Autodesk Fusion 360 part; units mm, degrees
(part 2 of 3)
extrude "Left inlet bore" cut sketch "Left inlet bore sketch" along normal blind 20.5 bodies 7 in component "06 Gas fitting envelopes TBD"
ref_plane "WorkPlane1" through (0, 0, 3.3) normal (0, 0, 1) x (1, 0, 0) in component "07 Guition 4.3in envelope — depth TBD"
sketch "Guition module envelope sketch" plane through (0, 0, 3.3) normal (0, 0, 1) x (1, 0, 0) in component "07 Guition 4.3in envelope — depth TBD"
  line L0 (-34.705, 10) -> (34.705, 10)
  line L1 (34.705, 10) -> (34.705, 127.01)
  line L2 (34.705, 127.01) -> (-34.705, 127.01)
  line L3 (-34.705, 127.01) -> (-34.705, 10)
  dimension "d549" = 34.705
  dimension "d550" = 10
  dimension "d551" = 69.41
  dimension "d552" = 117.01
  constraint horizontal L0
  constraint vertical L1
  constraint horizontal L2
  constraint vertical L3
  measures "d549" horizontal distance of origin L0.start
  measures "d550" vertical distance of origin L0.start
  measures "d551" horizontal distance of L0.start L0.end
  measures "d552" vertical distance of L0.end L1.end
extrude "Guition module envelope" add sketch "Guition module envelope sketch" along normal blind 13.8 separate body makes body 8 in component "07 Guition 4.3in envelope — depth TBD"
ref_plane "WorkPlane1" through (0, 0, 3.2) normal (0, 0, 1) x (1, 0, 0) in component "08 Active display reference"
sketch "4.3in active screen sketch" plane through (0, 0, 3.2) normal (0, 0, 1) x (1, 0, 0) in component "08 Active display reference"
  line L0 (-28.08, 21.705) -> (28.08, 21.705)
  line L1 (28.08, 21.705) -> (28.08, 115.305)
  line L2 (28.08, 115.305) -> (-28.08, 115.305)
  line L3 (-28.08, 115.305) -> (-28.08, 21.705)
  dimension "d557" = 28.08
  dimension "d558" = 21.705
  dimension "d559" = 56.16
  dimension "d560" = 93.6
  constraint horizontal L0
  constraint vertical L1
  constraint horizontal L2
  constraint vertical L3
  measures "d557" horizontal distance of origin L0.start
  measures "d558" vertical distance of origin L0.start
  measures "d559" horizontal distance of L0.start L0.end
  measures "d560" vertical distance of L0.end L1.end
extrude "4.3in active screen" add sketch "4.3in active screen sketch" along normal blind 0.1 separate body makes body 9 in component "08 Active display reference"
ref_plane "WorkPlane1" through (0, 0, 19) normal (0, 0, 1) x (1, 0, 0) in component "09 Removable electronics carrier"
sketch "Carrier side rail sketch" plane through (0, 0, 19) normal (0, 0, 1) x (1, 0, 0) in component "09 Removable electronics carrier"
  line L0 (-35, 10) -> (-32, 10)
  line L1 (-32, 10) -> (-32, 127)
  line L2 (-32, 127) -> (-35, 127)
  line L3 (-35, 127) -> (-35, 10)
  dimension "d565" = 35
  dimension "d566" = 10
  dimension "d567" = 3
  dimension "d568" = 117
  constraint horizontal L0
  constraint vertical L1
  constraint horizontal L2
  constraint vertical L3
  measures "d565" horizontal distance of origin L0.start
  measures "d566" vertical distance of origin L0.start
  measures "d567" horizontal distance of L0.start L0.end
  measures "d568" vertical distance of L0.end L1.end
extrude "Carrier side rail" add sketch "Carrier side rail sketch" along normal blind 3 separate body makes body 10 in component "09 Removable electronics carrier"
ref_plane "WorkPlane2" through (0, 0, 19) normal (0, 0, 1) x (1, 0, 0) in component "09 Removable electronics carrier"
sketch "Carrier side rail sketch (1)" plane through (0, 0, 19) normal (0, 0, 1) x (1, 0, 0) in component "09 Removable electronics carrier"
  line L0 (32, 10) -> (35, 10)
  line L1 (35, 10) -> (35, 127)
  line L2 (35, 127) -> (32, 127)
  line L3 (32, 127) -> (32, 10)
  dimension "d573" = 32
  dimension "d574" = 10
  dimension "d575" = 3
  dimension "d576" = 117
  constraint horizontal L0
  constraint vertical L1
  constraint horizontal L2
  constraint vertical L3
  measures "d573" horizontal distance of origin L0.start
  measures "d574" vertical distance of origin L0.start
  measures "d575" horizontal distance of L0.start L0.end
  measures "d576" vertical distance of L0.end L1.end
extrude "Carrier side rail (1)" add sketch "Carrier side rail sketch (1)" along normal blind 3 separate body makes body 11 in component "09 Removable electronics carrier"
ref_plane "WorkPlane3" through (0, 0, 19) normal (0, 0, 1) x (1, 0, 0) in component "09 Removable electronics carrier"
sketch "Carrier top crossbar sketch" plane through (0, 0, 19) normal (0, 0, 1) x (1, 0, 0) in component "09 Removable electronics carrier"
  line L0 (-35, 124) -> (35, 124)
  line L1 (35, 124) -> (35, 127)
  line L2 (35, 127) -> (-35, 127)
  line L3 (-35, 127) -> (-35, 124)
  dimension "d581" = 35
  dimension "d582" = 124
  dimension "d583" = 70
  dimension "d584" = 3
  constraint horizontal L0
  constraint vertical L1
  constraint horizontal L2
  constraint vertical L3
  measures "d581" horizontal distance of origin L0.start
  measures "d582" vertical distance of origin L0.start
  measures "d583" horizontal distance of L0.start L0.end
  measures "d584" vertical distance of L0.end L1.end
extrude "Carrier top crossbar" add sketch "Carrier top crossbar sketch" along normal blind 3 bodies 10 11 in component "09 Removable electronics carrier"
ref_plane "WorkPlane4" through (0, 0, 19) normal (0, 0, 1) x (1, 0, 0) in component "09 Removable electronics carrier"
sketch "Carrier middle crossbar sketch" plane through (0, 0, 19) normal (0, 0, 1) x (1, 0, 0) in component "09 Removable electronics carrier"
  line L0 (-35, 87) -> (35, 87)
  line L1 (35, 87) -> (35, 90)
  line L2 (35, 90) -> (-35, 90)
  line L3 (-35, 90) -> (-35, 87)
  dimension "d589" = 35
  dimension "d590" = 87
  dimension "d591" = 70
  dimension "d592" = 3
  constraint horizontal L0
  constraint vertical L1
  constraint horizontal L2
  constraint vertical L3
  measures "d589" horizontal distance of origin L0.start
  measures "d590" vertical distance of origin L0.start
  measures "d591" horizontal distance of L0.start L0.end
  measures "d592" vertical distance of L0.end L1.end
extrude "Carrier middle crossbar" add sketch "Carrier middle crossbar sketch" along normal blind 3 bodies 10 in component "09 Removable electronics carrier"
ref_plane "WorkPlane5" through (0, 0, 19) normal (0, 0, 1) x (1, 0, 0) in component "09 Removable electronics carrier"
sketch "Carrier mounting foot sketch" plane through (0, 0, 19) normal (0, 0, 1) x (1, 0, 0) in component "09 Removable electronics carrier"
  line L0 (-41, 17) -> (-32, 17)
  line L1 (-32, 17) -> (-32, 23)
  line L2 (-32, 23) -> (-41, 23)
  line L3 (-41, 23) -> (-41, 17)
  dimension "d597" = 41
  dimension "d598" = 17
  dimension "d599" = 9
  dimension "d600" = 6
  constraint horizontal L0
  constraint vertical L1
  constraint horizontal L2
  constraint vertical L3
  measures "d597" horizontal distance of origin L0.start
  measures "d598" vertical distance of origin L0.start
  measures "d599" horizontal distance of L0.start L0.end
  measures "d600" vertical distance of L0.end L1.end
extrude "Carrier mounting foot" add sketch "Carrier mounting foot sketch" along normal blind 3 bodies 10 in component "09 Removable electronics carrier"
ref_plane "WorkPlane6" through (0, 0, 18.9) normal (0, 0, 1) x (1, 0, 0) in component "09 Removable electronics carrier"
sketch "Carrier M3 clearance sketch" plane through (0, 0, 18.9) normal (0, 0, 1) x (1, 0, 0) in component "09 Removable electronics carrier"
  circle A0 centre (-38, 20) radius 1.7
  dimension "d605" = 38
  dimension "d606" = 20
  dimension "d607" = 1.7
  measures "d605" horizontal distance of origin A0.centre
  measures "d606" vertical distance of origin A0.centre
  measures "d607" radius of A0
extrude "Carrier M3 clearance" cut sketch "Carrier M3 clearance sketch" along normal blind 3.2 bodies 10 in component "09 Removable electronics carrier"
ref_plane "WorkPlane33" through (0, 0, 3) normal (0, 0, 1) x (1, 0, 0) in component "01 Main housing"
sketch "Carrier support sketch" plane through (0, 0, 3) normal (0, 0, 1) x (1, 0, 0) in component "01 Main housing"
  circle A0 centre (-38, 20) radius 3
  dimension "d612" = 38
  dimension "d613" = 20
  dimension "d614" = 3
  measures "d612" horizontal distance of origin A0.centre
  measures "d613" vertical distance of origin A0.centre
  measures "d614" radius of A0
extrude "Carrier support" add sketch "Carrier support sketch" along normal blind 16 bodies 1 in component "01 Main housing"
ref_plane "WorkPlane34" through (0, 0, 14) normal (0, 0, 1) x (1, 0, 0) in component "01 Main housing"
sketch "Carrier support pilot sketch" plane through (0, 0, 14) normal (0, 0, 1) x (1, 0, 0) in component "01 Main housing"
  circle A0 centre (-38, 20) radius 2.1
  dimension "d619" = 38
  dimension "d620" = 20
  dimension "d621" = 2.1
  measures "d619" horizontal distance of origin A0.centre
  measures "d620" vertical distance of origin A0.centre
  measures "d621" radius of A0
extrude "Carrier support pilot" cut sketch "Carrier support pilot sketch" along normal blind 5.1 bodies 1 in component "01 Main housing"
ref_plane "WorkPlane7" through (0, 0, 19) normal (0, 0, 1) x (1, 0, 0) in component "09 Removable electronics carrier"
sketch "Carrier mounting foot sketch (1)" plane through (0, 0, 19) normal (0, 0, 1) x (1, 0, 0) in component "09 Removable electronics carrier"
  line L0 (-41, 121) -> (-32, 121)
  line L1 (-32, 121) -> (-32, 127)
  line L2 (-32, 127) -> (-41, 127)
  line L3 (-41, 127) -> (-41, 121)
  dimension "d626" = 41
  dimension "d627" = 121
  dimension "d628" = 9
  dimension "d629" = 6
  constraint horizontal L0
  constraint vertical L1
  constraint horizontal L2
  constraint vertical L3
  measures "d626" horizontal distance of origin L0.start
  measures "d627" vertical distance of origin L0.start
  measures "d628" horizontal distance of L0.start L0.end
  measures "d629" vertical distance of L0.end L1.end
extrude "Carrier mounting foot (1)" add sketch "Carrier mounting foot sketch (1)" along normal blind 3 bodies 10 in component "09 Removable electronics carrier"
ref_plane "WorkPlane8" through (0, 0, 18.9) normal (0, 0, 1) x (1, 0, 0) in component "09 Removable electronics carrier"
sketch "Carrier M3 clearance sketch (1)" plane through (0, 0, 18.9) normal (0, 0, 1) x (1, 0, 0) in component "09 Removable electronics carrier"
  circle A0 centre (-38, 124) radius 1.7
  dimension "d634" = 38
  dimension "d635" = 124
  dimension "d636" = 1.7
  measures "d634" horizontal distance of origin A0.centre
  measures "d635" vertical distance of origin A0.centre
  measures "d636" radius of A0
extrude "Carrier M3 clearance (1)" cut sketch "Carrier M3 clearance sketch (1)" along normal blind 3.2 bodies 10 in component "09 Removable electronics carrier"
ref_plane "WorkPlane35" through (0, 0, 3) normal (0, 0, 1) x (1, 0, 0) in component "01 Main housing"
sketch "Carrier support sketch (1)" plane through (0, 0, 3) normal (0, 0, 1) x (1, 0, 0) in component "01 Main housing"
  circle A0 centre (-38, 124) radius 3
  dimension "d641" = 38
  dimension "d642" = 124
  dimension "d643" = 3
  measures "d641" horizontal distance of origin A0.centre
  measures "d642" vertical distance of origin A0.centre
  measures "d643" radius of A0
extrude "Carrier support (1)" add sketch "Carrier support sketch (1)" along normal blind 16 bodies 1 in component "01 Main housing"
ref_plane "WorkPlane36" through (0, 0, 14) normal (0, 0, 1) x (1, 0, 0) in component "01 Main housing"
sketch "Carrier support pilot sketch (1)" plane through (0, 0, 14) normal (0, 0, 1) x (1, 0, 0) in component "01 Main housing"
  circle A0 centre (-38, 124) radius 2.1
  dimension "d648" = 38
  dimension "d649" = 124
  dimension "d650" = 2.1
  measures "d648" horizontal distance of origin A0.centre
  measures "d649" vertical distance of origin A0.centre
  measures "d650" radius of A0
extrude "Carrier support pilot (1)" cut sketch "Carrier support pilot sketch (1)" along normal blind 5.1 bodies 1 in component "01 Main housing"
ref_plane "WorkPlane9" through (0, 0, 19) normal (0, 0, 1) x (1, 0, 0) in component "09 Removable electronics carrier"
sketch "Carrier mounting foot sketch (2)" plane through (0, 0, 19) normal (0, 0, 1) x (1, 0, 0) in component "09 Removable electronics carrier"
  line L0 (32, 17) -> (41, 17)
  line L1 (41, 17) -> (41, 23)
  line L2 (41, 23) -> (32, 23)
  line L3 (32, 23) -> (32, 17)
  dimension "d655" = 32
  dimension "d656" = 17
  dimension "d657" = 9
  dimension "d658" = 6
  constraint horizontal L0
  constraint vertical L1
  constraint horizontal L2
  constraint vertical L3
  measures "d655" horizontal distance of origin L0.start
  measures "d656" vertical distance of origin L0.start
  measures "d657" horizontal distance of L0.start L0.end
  measures "d658" vertical distance of L0.end L1.end
extrude "Carrier mounting foot (2)" add sketch "Carrier mounting foot sketch (2)" along normal blind 3 bodies 10 in component "09 Removable electronics carrier"
ref_plane "WorkPlane10" through (0, 0, 18.9) normal (0, 0, 1) x (1, 0, 0) in component "09 Removable electronics carrier"
sketch "Carrier M3 clearance sketch (2)" plane through (0, 0, 18.9) normal (0, 0, 1) x (1, 0, 0) in component "09 Removable electronics carrier"
  circle A0 centre (38, 20) radius 1.7
  dimension "d663" = 38
  dimension "d664" = 20
  dimension "d665" = 1.7
  measures "d663" horizontal distance of origin A0.centre
  measures "d664" vertical distance of origin A0.centre
  measures "d665" radius of A0
extrude "Carrier M3 clearance (2)" cut sketch "Carrier M3 clearance sketch (2)" along normal blind 3.2 bodies 10 in component "09 Removable electronics carrier"
ref_plane "WorkPlane37" through (0, 0, 3) normal (0, 0, 1) x (1, 0, 0) in component "01 Main housing"
sketch "Carrier support sketch (2)" plane through (0, 0, 3) normal (0, 0, 1) x (1, 0, 0) in component "01 Main housing"
  circle A0 centre (38, 20) radius 3
  dimension "d670" = 38
  dimension "d671" = 20
  dimension "d672" = 3
  measures "d670" horizontal distance of origin A0.centre
  measures "d671" vertical distance of origin A0.centre
  measures "d672" radius of A0
extrude "Carrier support (2)" add sketch "Carrier support sketch (2)" along normal blind 16 bodies 1 in component "01 Main housing"
ref_plane "WorkPlane38" through (0, 0, 14) normal (0, 0, 1) x (1, 0, 0) in component "01 Main housing"
sketch "Carrier support pilot sketch (2)" plane through (0, 0, 14) normal (0, 0, 1) x (1, 0, 0) in component "01 Main housing"
  circle A0 centre (38, 20) radius 2.1
  dimension "d677" = 38
  dimension "d678" = 20
  dimension "d679" = 2.1
  measures "d677" horizontal distance of origin A0.centre
  measures "d678" vertical distance of origin A0.centre
  measures "d679" radius of A0
extrude "Carrier support pilot (2)" cut sketch "Carrier support pilot sketch (2)" along normal blind 5.1 bodies 1 in component "01 Main housing"
ref_plane "WorkPlane11" through (0, 0, 19) normal (0, 0, 1) x (1, 0, 0) in component "09 Removable electronics carrier"
sketch "Carrier mounting foot sketch (3)" plane through (0, 0, 19) normal (0, 0, 1) x (1, 0, 0) in component "09 Removable electronics carrier"
  line L0 (32, 121) -> (41, 121)
  line L1 (41, 121) -> (41, 127)
  line L2 (41, 127) -> (32, 127)
  line L3 (32, 127) -> (32, 121)
  dimension "d684" = 32
  dimension "d685" = 121
  dimension "d686" = 9
  dimension "d687" = 6
  constraint horizontal L0
  constraint vertical L1
  constraint horizontal L2
  constraint vertical L3
  measures "d684" horizontal distance of origin L0.start
  measures "d685" vertical distance of origin L0.start
  measures "d686" horizontal distance of L0.start L0.end
  measures "d687" vertical distance of L0.end L1.end
extrude "Carrier mounting foot (3)" add sketch "Carrier mounting foot sketch (3)" along normal blind 3 bodies 10 in component "09 Removable electronics carrier"
ref_plane "WorkPlane12" through (0, 0, 18.9) normal (0, 0, 1) x (1, 0, 0) in component "09 Removable electronics carrier"
sketch "Carrier M3 clearance sketch (3)" plane through (0, 0, 18.9) normal (0, 0, 1) x (1, 0, 0) in component "09 Removable electronics carrier"
  circle A0 centre (38, 124) radius 1.7
  dimension "d692" = 38
  dimension "d693" = 124
  dimension "d694" = 1.7
  measures "d692" horizontal distance of origin A0.centre
  measures "d693" vertical distance of origin A0.centre
  measures "d694" radius of A0
extrude "Carrier M3 clearance (3)" cut sketch "Carrier M3 clearance sketch (3)" along normal blind 3.2 bodies 10 in component "09 Removable electronics carrier"
ref_plane "WorkPlane39" through (0, 0, 3) normal (0, 0, 1) x (1, 0, 0) in component "01 Main housing"
sketch "Carrier support sketch (3)" plane through (0, 0, 3) normal (0, 0, 1) x (1, 0, 0) in component "01 Main housing"
  circle A0 centre (38, 124) radius 3
  dimension "d699" = 38
  dimension "d700" = 124
  dimension "d701" = 3
  measures "d699" horizontal distance of origin A0.centre
  measures "d700" vertical distance of origin A0.centre
  measures "d701" radius of A0
extrude "Carrier support (3)" add sketch "Carrier support sketch (3)" along normal blind 16 bodies 1 in component "01 Main housing"
ref_plane "WorkPlane40" through (0, 0, 14) normal (0, 0, 1) x (1, 0, 0) in component "01 Main housing"
sketch "Carrier support pilot sketch (3)" plane through (0, 0, 14) normal (0, 0, 1) x (1, 0, 0) in component "01 Main housing"
  circle A0 centre (38, 124) radius 2.1
  dimension "d706" = 38
  dimension "d707" = 124
  dimension "d708" = 2.1
  measures "d706" horizontal distance of origin A0.centre
  measures "d707" vertical distance of origin A0.centre
  measures "d708" radius of A0
extrude "Carrier support pilot (3)" cut sketch "Carrier support pilot sketch (3)" along normal blind 5.1 bodies 1 in component "01 Main housing"
ref_plane "WorkPlane1" through (0, 0, 23) normal (0, 0, 1) x (1, 0, 0) in component "10 Future PCB and component envelope TBD"
sketch "Sketch1 (2)" plane through (0, 0, 23) normal (0, 0, 1) x (1, 0, 0) in component "10 Future PCB and component envelope TBD"
  line L0 (-32, 14) -> (32, 14)
  line L1 (32, 14) -> (32, 122)
  line L2 (32, 122) -> (-32, 122)
  line L3 (-32, 122) -> (-32, 14)
  dimension "d713" = 32
  dimension "d714" = 14
  dimension "d715" = 64
  dimension "d716" = 108
  constraint horizontal L0
  constraint vertical L1
  constraint horizontal L2
  constraint vertical L3
  measures "d713" horizontal distance of origin L0.start
  measures "d714" vertical distance of origin L0.start
  measures "d715" horizontal distance of L0.start L0.end
  measures "d716" vertical distance of L0.end L1.end
extrude "Future PCB envelope — not routed KiCad board" add sketch "Sketch1 (2)" along normal blind 1.6 separate body makes body 12 in component "10 Future PCB and component envelope TBD"
ref_plane "WorkPlane2" through (0, 0, 18.5) normal (0, 0, 1) x (1, 0, 0) in component "10 Future PCB and component envelope TBD"
sketch "Lower PCB component allowance sketch" plane through (0, 0, 18.5) normal (0, 0, 1) x (1, 0, 0) in component "10 Future PCB and component envelope TBD"
  line L0 (-27, 18) -> (27, 18)
  line L1 (27, 18) -> (27, 84)
  line L2 (27, 84) -> (-27, 84)
  line L3 (-27, 84) -> (-27, 18)
  dimension "d721" = 27
  dimension "d722" = 18
  dimension "d723" = 54
  dimension "d724" = 66
  constraint horizontal L0
  constraint vertical L1
  constraint horizontal L2
  constraint vertical L3
  measures "d721" horizontal distance of origin L0.start
  measures "d722" vertical distance of origin L0.start
  measures "d723" horizontal distance of L0.start L0.end
  measures "d724" vertical distance of L0.end L1.end
extrude "Lower PCB component allowance" add sketch "Lower PCB component allowance sketch" along normal blind 4.5 separate body makes body 13 in component "10 Future PCB and component envelope TBD"
ref_plane "WorkPlane3" through (0, 0, 18.5) normal (0, 0, 1) x (1, 0, 0) in component "10 Future PCB and component envelope TBD"
sketch "Upper PCB component allowance sketch" plane through (0, 0, 18.5) normal (0, 0, 1) x (1, 0, 0) in component "10 Future PCB and component envelope TBD"
  line L0 (-27, 93) -> (27, 93)
  line L1 (27, 93) -> (27, 121)
  line L2 (27, 121) -> (-27, 121)
  line L3 (-27, 121) -> (-27, 93)
  dimension "d729" = 27
  dimension "d730" = 93
  dimension "d731" = 54
  dimension "d732" = 28
  constraint horizontal L0
  constraint vertical L1
  constraint horizontal L2
  constraint vertical L3
  measures "d729" horizontal distance of origin L0.start
  measures "d730" vertical distance of origin L0.start
  measures "d731" horizontal distance of L0.start L0.end
  measures "d732" vertical distance of L0.end L1.end
extrude "Upper PCB component allowance" add sketch "Upper PCB component allowance sketch" along normal blind 4.5 separate body makes body 14 in component "10 Future PCB and component envelope TBD"
ref_plane "WorkPlane1" through (0, 0, 27) normal (0, 0, 1) x (1, 0, 0) in component "11 Protected FMA holder envelope TBD"
sketch "FMA holder envelope TBD sketch" plane through (0, 0, 27) normal (0, 0, 1) x (1, 0, 0) in component "11 Protected FMA holder envelope TBD"
  line L0 (-22, 12) -> (22, 12)
  line L1 (22, 12) -> (22, 88)
  line L2 (22, 88) -> (-22, 88)
  line L3 (-22, 88) -> (-22, 12)
  dimension "d737" = 22
  dimension "d738" = 12
  dimension "d739" = 44
  dimension "d740" = 76
  constraint horizontal L0
  constraint vertical L1
  constraint horizontal L2
  constraint vertical L3
  measures "d737" horizontal distance of origin L0.start
  measures "d738" vertical distance of origin L0.start
  measures "d739" horizontal distance of L0.start L0.end
  measures "d740" vertical distance of L0.end L1.end
extrude "FMA holder envelope TBD" add sketch "FMA holder envelope TBD sketch" along normal blind 28 separate body makes body 15 in component "11 Protected FMA holder envelope TBD"
ref_plane "WorkPlane2" through (0, 0, 29) normal (0, 0, 1) x (1, 0, 0) in component "11 Protected FMA holder envelope TBD"
sketch "Two-cell cavity envelope sketch" plane through (0, 0, 29) normal (0, 0, 1) x (1, 0, 0) in component "11 Protected FMA holder envelope TBD"
  line L0 (-20, 16) -> (20, 16)
  line L1 (20, 16) -> (20, 84)
  line L2 (20, 84) -> (-20, 84)
  line L3 (-20, 84) -> (-20, 16)
  dimension "d745" = 20
  dimension "d746" = 16
  dimension "d747" = 40
  dimension "d748" = 68
  constraint horizontal L0
  constraint vertical L1
  constraint horizontal L2
  constraint vertical L3
  measures "d745" horizontal distance of origin L0.start
  measures "d746" vertical distance of origin L0.start
  measures "d747" horizontal distance of L0.start L0.end
  measures "d748" vertical distance of L0.end L1.end
extrude "Two-cell cavity envelope" cut sketch "Two-cell cavity envelope sketch" along normal blind 27 bodies 15 in component "11 Protected FMA holder envelope TBD"
ref_plane "WorkPlane1" through (0, 17, 0) normal (0, 1, 0) x (0, 0, 1) in component "12 Two 18650 cell envelopes"
sketch "18650 envelope" plane through (0, 17, 0) normal (0, 1, 0) x (1, 0, 0) in component "12 Two 18650 cell envelopes"
  circle A0 centre (-10, -39) radius 9.3
  dimension "d753" = 10
  dimension "d754" = 39
  dimension "d755" = 9.3
  measures "d753" horizontal distance of origin A0.centre
  measures "d754" vertical distance of origin A0.centre
  measures "d755" radius of A0
extrude "18650 cell envelope" add sketch "18650 envelope" along normal blind 65.5 separate body makes body 16 in component "12 Two 18650 cell envelopes"
ref_plane "WorkPlane2" through (0, 17, 0) normal (0, 1, 0) x (0, 0, 1) in component "12 Two 18650 cell envelopes"
sketch "18650 envelope (1)" plane through (0, 17, 0) normal (0, 1, 0) x (1, 0, 0) in component "12 Two 18650 cell envelopes"
  circle A0 centre (10, -39) radius 9.3
  dimension "d760" = 10
  dimension "d761" = 39
  dimension "d762" = 9.3
  measures "d760" horizontal distance of origin A0.centre
  measures "d761" vertical distance of origin A0.centre
  measures "d762" radius of A0
extrude "18650 cell envelope (1)" add sketch "18650 envelope (1)" along normal blind 65.5 separate body makes body 17 in component "12 Two 18650 cell envelopes"
ref_plane "WorkPlane1" through (0, 0, 38) normal (0, 0, 1) x (1, 0, 0) in component "13 Battery plug and cable clearance TBD"
sketch "RCY BEC disconnect clearance sketch" plane through (0, 0, 38) normal (0, 0, 1) x (1, 0, 0) in component "13 Battery plug and cable clearance TBD"
  line L0 (23, 18) -> (33, 18)
  line L1 (33, 18) -> (33, 40)
  line L2 (33, 40) -> (23, 40)
  line L3 (23, 40) -> (23, 18)
  dimension "d767" = 23
  dimension "d768" = 18
  dimension "d769" = 10
  dimension "d770" = 22
  constraint horizontal L0
  constraint vertical L1
  constraint horizontal L2
  constraint vertical L3
  measures "d767" horizontal distance of origin L0.start
  measures "d768" vertical distance of origin L0.start
  measures "d769" horizontal distance of L0.start L0.end
  measures "d770" vertical distance of L0.end L1.end
extrude "RCY BEC disconnect clearance" add sketch "RCY BEC disconnect clearance sketch" along normal blind 14 separate body makes body 18 in component "13 Battery plug and cable clearance TBD"
ref_plane "WorkPlane1" through (44.5, 0, 0) normal (1, 0, 0) x (0, 1, 0) in component "14 Supported USB-C mounting insert TBD"
sketch "Replaceable USB insert sketch" plane through (44.5, 0, 0) normal (1, 0, 0) x (0, 0, -1) in component "14 Supported USB-C mounting insert TBD"
  line L0 (-41.75, 58.25) -> (-26.25, 58.25)
  line L1 (-26.25, 58.25) -> (-26.25, 77.75)
  line L2 (-26.25, 77.75) -> (-41.75, 77.75)
  line L3 (-41.75, 77.75) -> (-41.75, 58.25)
  dimension "d775" = 41.75
  dimension "d776" = 58.25
  dimension "d777" = 15.5
  dimension "d778" = 19.5
  constraint horizontal L0
  constraint vertical L1
  constraint horizontal L2
  constraint vertical L3
  measures "d775" horizontal distance of origin L0.start
  measures "d776" vertical distance of origin L0.start
  measures "d777" horizontal distance of L0.start L0.end
  measures "d778" vertical distance of L0.end L1.end
extrude "Replaceable USB insert" add sketch "Replaceable USB insert sketch" along normal blind 3 separate body makes body 19 in component "14 Supported USB-C mounting insert TBD"
ref_plane "WorkPlane2" through (42.5, 0, 0) normal (1, 0, 0) x (0, 1, 0) in component "14 Supported USB-C mounting insert TBD"
sketch "USB interior backing flange sketch" plane through (42.5, 0, 0) normal (1, 0, 0) x (0, 0, -1) in component "14 Supported USB-C mounting insert TBD"
  line L0 (-44, 56) -> (-24, 56)
  line L1 (-24, 56) -> (-24, 80)
  line L2 (-24, 80) -> (-44, 80)
  line L3 (-44, 80) -> (-44, 56)
  dimension "d783" = 44
  dimension "d784" = 56
  dimension "d785" = 20
  dimension "d786" = 24
  constraint horizontal L0
  constraint vertical L1
  constraint horizontal L2
  constraint vertical L3
  measures "d783" horizontal distance of origin L0.start
  measures "d784" vertical distance of origin L0.start
  measures "d785" horizontal distance of L0.start L0.end
  measures "d786" vertical distance of L0.end L1.end
extrude "USB interior backing flange" add sketch "USB interior backing flange sketch" along normal blind 2 separate body makes body 20 in component "14 Supported USB-C mounting insert TBD"
ref_plane "WorkPlane3" through (42.4, 0, 0) normal (1, 0, 0) x (0, 1, 0) in component "14 Supported USB-C mounting insert TBD"
sketch "Sketch3 (2)" plane through (42.4, 0, 0) normal (1, 0, 0) x (0, 0, -1) in component "14 Supported USB-C mounting insert TBD"
  line L0 (-35.93, 63.18) -> (-32.07, 63.18)
  line L1 (-32.07, 63.18) -> (-32.07, 72.82)
  line L2 (-32.07, 72.82) -> (-35.93, 72.82)
  line L3 (-35.93, 72.82) -> (-35.93, 63.18)
  dimension "d791" = 35.93
  dimension "d792" = 63.18
  dimension "d793" = 3.86
  dimension "d794" = 9.64
  constraint horizontal L0
  constraint vertical L1
  constraint horizontal L2
  constraint vertical L3
  measures "d791" horizontal distance of origin L0.start
  measures "d792" vertical distance of origin L0.start
  measures "d793" horizontal distance of L0.start L0.end
  measures "d794" vertical distance of L0.end L1.end
extrude "USB aperture envelope — GCT step profile TBD" cut sketch "Sketch3 (2)" along normal blind 5.2 bodies 19 in component "14 Supported USB-C mounting insert TBD"
ref_plane "WorkPlane4" through (42.4, 0, 0) normal (1, 0, 0) x (0, 1, 0) in component "14 Supported USB-C mounting insert TBD"
sketch "USB backing aperture sketch" plane through (42.4, 0, 0) normal (1, 0, 0) x (0, 0, -1) in component "14 Supported USB-C mounting insert TBD"
  line L0 (-35.93, 63.18) -> (-32.07, 63.18)
  line L1 (-32.07, 63.18) -> (-32.07, 72.82)
  line L2 (-32.07, 72.82) -> (-35.93, 72.82)
  line L3 (-35.93, 72.82) -> (-35.93, 63.18)
  dimension "d799" = 35.93
  dimension "d800" = 63.18
  dimension "d801" = 3.86
  dimension "d802" = 9.64
  constraint horizontal L0
  constraint vertical L1
  constraint horizontal L2
  constraint vertical L3
  measures "d799" horizontal distance of origin L0.start
  measures "d800" vertical distance of origin L0.start
  measures "d801" horizontal distance of L0.start L0.end
  measures "d802" vertical distance of L0.end L1.end
extrude "USB backing aperture" cut sketch "USB backing aperture sketch" along normal blind 2.2 bodies 20 in component "14 Supported USB-C mounting insert TBD"
ref_plane "WorkPlane1" through (0, 0, 33.7) normal (0, 0, 1) x (1, 0, 0) in component "15 USB daughterboard envelope 0.60mm"
sketch "Sketch1 (3)" plane through (0, 0, 33.7) normal (0, 0, 1) x (1, 0, 0) in component "15 USB daughterboard envelope 0.60mm"
  line L0 (29, 60) -> (41, 60)
  line L1 (41, 60) -> (41, 76)
  line L2 (41, 76) -> (29, 76)
  line L3 (29, 76) -> (29, 60)
  dimension "d807" = 29
  dimension "d808" = 60
  dimension "d809" = 12
  dimension "d810" = 16
  constraint horizontal L0
  constraint vertical L1
  constraint horizontal L2
  constraint vertical L3
  measures "d807" horizontal distance of origin L0.start
  measures "d808" vertical distance of origin L0.start
  measures "d809" horizontal distance of L0.start L0.end
  measures "d810" vertical distance of L0.end L1.end
extrude "USB daughterboard — layout TBD" add sketch "Sketch1 (3)" along normal blind 0.6 separate body makes body 21 in component "15 USB daughterboard envelope 0.60mm"
ref_plane "WorkPlane2" through (0, 0, 32.5) normal (0, 0, 1) x (1, 0, 0) in component "15 USB daughterboard envelope 0.60mm"
sketch "GCT connector envelope TBD sketch" plane through (0, 0, 32.5) normal (0, 0, 1) x (1, 0, 0) in component "15 USB daughterboard envelope 0.60mm"
  line L0 (34, 63.5) -> (47.5, 63.5)
  line L1 (47.5, 63.5) -> (47.5, 72.5)
  line L2 (47.5, 72.5) -> (34, 72.5)
  line L3 (34, 72.5) -> (34, 63.5)
  dimension "d815" = 34
  dimension "d816" = 63.5
  dimension "d817" = 13.5
  dimension "d818" = 9
  constraint horizontal L0
  constraint vertical L1
  constraint horizontal L2
  constraint vertical L3
  measures "d815" horizontal distance of origin L0.start
  measures "d816" vertical distance of origin L0.start
  measures "d817" horizontal distance of L0.start L0.end
  measures "d818" vertical distance of L0.end L1.end
extrude "GCT connector envelope TBD" add sketch "GCT connector envelope TBD sketch" along normal blind 3 separate body makes body 22 in component "15 USB daughterboard envelope 0.60mm"
ref_plane "WorkPlane5" through (0, 0, 31.7) normal (0, 0, 1) x (1, 0, 0) in component "14 Supported USB-C mounting insert TBD"
sketch "USB board support ledge sketch" plane through (0, 0, 31.7) normal (0, 0, 1) x (1, 0, 0) in component "14 Supported USB-C mounting insert TBD"
  line L0 (29, 60) -> (42.5, 60)
  line L1 (42.5, 60) -> (42.5, 62)
  line L2 (42.5, 62) -> (29, 62)
  line L3 (29, 62) -> (29, 60)
  dimension "d823" = 29
  dimension "d824" = 60
  dimension "d825" = 13.5
  dimension "d826" = 2
  constraint horizontal L0
  constraint vertical L1
  constraint horizontal L2
  constraint vertical L3
  measures "d823" horizontal distance of origin L0.start
  measures "d824" vertical distance of origin L0.start
  measures "d825" horizontal distance of L0.start L0.end
  measures "d826" vertical distance of L0.end L1.end
extrude "USB board support ledge" add sketch "USB board support ledge sketch" along normal blind 2 separate body makes body 23 in component "14 Supported USB-C mounting insert TBD"
ref_plane "WorkPlane6" through (0, 0, 31.7) normal (0, 0, 1) x (1, 0, 0) in component "14 Supported USB-C mounting insert TBD"
sketch "USB board support ledge sketch (1)" plane through (0, 0, 31.7) normal (0, 0, 1) x (1, 0, 0) in component "14 Supported USB-C mounting insert TBD"
  line L0 (29, 74) -> (42.5, 74)
  line L1 (42.5, 74) -> (42.5, 76)
  line L2 (42.5, 76) -> (29, 76)
  line L3 (29, 76) -> (29, 74)
  dimension "d831" = 29
  dimension "d832" = 74
  dimension "d833" = 13.5
  dimension "d834" = 2
  constraint horizontal L0
  constraint vertical L1
  constraint horizontal L2
  constraint vertical L3
  measures "d831" horizontal distance of origin L0.start
  measures "d832" vertical distance of origin L0.start
  measures "d833" horizontal distance of L0.start L0.end
  measures "d834" vertical distance of L0.end L1.end
extrude "USB board support ledge (1)" add sketch "USB board support ledge sketch (1)" along normal blind 2 separate body makes body 24 in component "14 Supported USB-C mounting insert TBD"
ref_plane "WorkPlane1" through (-47.5, 0, 0) normal (1, 0, 0) x (0, 1, 0) in component "16 Right momentary button envelope TBD"
sketch "12 mm button barrel envelope sketch" plane through (-47.5, 0, 0) normal (1, 0, 0) x (0, 0, -1) in component "16 Right momentary button envelope TBD"
  circle A0 centre (-42, 102) radius 5.8
  dimension "d840" = 102
  dimension "d841" = 5.8
  measures "d840" vertical distance of origin A0.centre
  measures "d841" radius of A0
extrude "12 mm button barrel envelope" add sketch "12 mm button barrel envelope sketch" along normal blind 18 separate body makes body 25 in component "16 Right momentary button envelope TBD"
ref_plane "WorkPlane2" through (-49, 0, 0) normal (1, 0, 0) x (0, 1, 0) in component "16 Right momentary button envelope TBD"
sketch "Power button bezel envelope sketch" plane through (-49, 0, 0) normal (1, 0, 0) x (0, 0, -1) in component "16 Right momentary button envelope TBD"
  circle A0 centre (-42, 102) radius 7
  dimension "d847" = 102
  dimension "d848" = 7
  measures "d847" vertical distance of origin A0.centre
  measures "d848" radius of A0
extrude "Power button bezel envelope" add sketch "Power button bezel envelope sketch" along normal blind 1.5 separate body makes body 26 in component "16 Right momentary button envelope TBD"
ref_plane "WorkPlane3" through (-29.5, 0, 0) normal (1, 0, 0) x (0, 1, 0) in component "16 Right momentary button envelope TBD"
sketch "Button terminal clearance TBD sketch" plane through (-29.5, 0, 0) normal (1, 0, 0) x (0, 0, -1) in component "16 Right momentary button envelope TBD"
  line L0 (-48, 96) -> (-36, 96)
  line L1 (-36, 96) -> (-36, 108)
  line L2 (-36, 108) -> (-48, 108)
  line L3 (-48, 108) -> (-48, 96)
  dimension "d853" = 48
  dimension "d854" = 96
  dimension "d855" = 12
  dimension "d856" = 12
  constraint horizontal L0
  constraint vertical L1
  constraint horizontal L2
  constraint vertical L3
  measures "d853" horizontal distance of origin L0.start
  measures "d854" vertical distance of origin L0.start
  measures "d855" horizontal distance of L0.start L0.end
  measures "d856" vertical distance of L0.end L1.end
extrude "Button terminal clearance TBD" add sketch "Button terminal clearance TBD sketch" along normal blind 7 separate body makes body 27 in component "16 Right momentary button envelope TBD"
ref_plane "WorkPlane1" through (0, 0, 48) normal (0, 0, 1) x (1, 0, 0) in component "18 Wiring route clearance envelopes"
sketch "Sensor loom route sketch" plane through (0, 0, 48) normal (0, 0, 1) x (1, 0, 0) in component "18 Wiring route clearance envelopes"
  line L0 (-5, 124) -> (5, 124)
  line L1 (5, 124) -> (5, 132)
  line L2 (5, 132) -> (-5, 132)
  line L3 (-5, 132) -> (-5, 124)
  dimension "d915" = 5
  dimension "d916" = 124
  dimension "d917" = 10
  dimension "d918" = 8
  constraint horizontal L0
  constraint vertical L1
  constraint horizontal L2
  constraint vertical L3
  measures "d915" horizontal distance of origin L0.start
  measures "d916" vertical distance of origin L0.start
  measures "d917" horizontal distance of L0.start L0.end
  measures "d918" vertical distance of L0.end L1.end
extrude "Sensor loom route" add sketch "Sensor loom route sketch" along normal blind 5 separate body makes body 28 in component "18 Wiring route clearance envelopes"
ref_plane "WorkPlane2" through (0, 0, 48) normal (0, 0, 1) x (1, 0, 0) in component "18 Wiring route clearance envelopes"
sketch "Main cable route sketch" plane through (0, 0, 48) normal (0, 0, 1) x (1, 0, 0) in component "18 Wiring route clearance envelopes"
  line L0 (26, 42) -> (32, 42)
  line L1 (32, 42) -> (32, 122)
  line L2 (32, 122) -> (26, 122)
  line L3 (26, 122) -> (26, 42)
  dimension "d923" = 26
  dimension "d924" = 42
  dimension "d925" = 6
  dimension "d926" = 80
  constraint horizontal L0
  constraint vertical L1
  constraint horizontal L2
  constraint vertical L3
  measures "d923" horizontal distance of origin L0.start
  measures "d924" vertical distance of origin L0.start
  measures "d925" horizontal distance of L0.start L0.end
  measures "d926" vertical distance of L0.end L1.end
extrude "Main cable route" add sketch "Main cable route sketch" along normal blind 5 separate body makes body 29 in component "18 Wiring route clearance envelopes"
ref_plane "WorkPlane3" through (0, 0, 33.6) normal (0, 0, 1) x (1, 0, 0) in component "15 USB daughterboard envelope 0.60mm"
sketch "USB straddle-mount board clearance TBD sketch" plane through (0, 0, 33.6) normal (0, 0, 1) x (1, 0, 0) in component "15 USB daughterboard envelope 0.60mm"
  line L0 (33.9, 63.4) -> (41.9, 63.4)
  line L1 (41.9, 63.4) -> (41.9, 72.6)
  line L2 (41.9, 72.6) -> (33.9, 72.6)
  line L3 (33.9, 72.6) -> (33.9, 63.4)
  dimension "d931" = 33.9
  dimension "d932" = 63.4
  dimension "d933" = 8
  dimension "d934" = 9.2
  constraint horizontal L0
  constraint vertical L1
  constraint horizontal L2
  constraint vertical L3
  measures "d931" horizontal distance of origin L0.start
  measures "d932" vertical distance of origin L0.start
  measures "d933" horizontal distance of L0.start L0.end
  measures "d934" vertical distance of L0.end L1.end
extrude "USB straddle-mount board clearance TBD" cut sketch "USB straddle-mount board clearance TBD sketch" along normal blind 0.8 bodies 21 in component "15 USB daughterboard envelope 0.60mm"
ref_plane "WorkPlane1" through (0, 0, 15.5) normal (0, 0, 1) x (1, 0, 0) in component "17 Chamber sensor envelopes TBD"
sketch "AO2 body diameter29.3 length31.75 sketch" plane through (0, 0, 15.5) normal (0, 0, 1) x (1, 0, 0) in component "17 Chamber sensor envelopes TBD"
  circle A0 centre (9, 153.5) radius 14.65
  dimension "d939" = 9
  dimension "d940" = 153.5
  dimension "d941" = 14.65
  measures "d939" horizontal distance of origin A0.centre
  measures "d940" vertical distance of origin A0.centre
  measures "d941" radius of A0
extrude "AO2 body diameter29.3 length31.75" add sketch "AO2 body diameter29.3 length31.75 sketch" along normal blind 31.75 separate body makes body 30 in component "17 Chamber sensor envelopes TBD"
ref_plane "WorkPlane2" through (0, 0, 9) normal (0, 0, 1) x (1, 0, 0) in component "17 Chamber sensor envelopes TBD"
sketch "Sketch2" plane through (0, 0, 9) normal (0, 0, 1) x (1, 0, 0) in component "17 Chamber sensor envelopes TBD"
  circle A0 centre (9, 153.5) radius 8
  dimension "d946" = 9
  dimension "d947" = 153.5
  dimension "d948" = 8
  measures "d946" horizontal distance of origin A0.centre
  measures "d947" vertical distance of origin A0.centre
  measures "d948" radius of A0
extrude "AO2 M16 neck envelope — no final thread" add sketch "Sketch2" along normal blind 6.5 separate body makes body 31 in component "17 Chamber sensor envelopes TBD"
ref_plane "WorkPlane3" through (0, 0, 47.25) normal (0, 0, 1) x (1, 0, 0) in component "17 Chamber sensor envelopes TBD"
sketch "AO2 connector and cable allowance sketch" plane through (0, 0, 47.25) normal (0, 0, 1) x (1, 0, 0) in component "17 Chamber sensor envelopes TBD"
  line L0 (4, 148.5) -> (14, 148.5)
  line L1 (14, 148.5) -> (14, 158.5)
  line L2 (14, 158.5) -> (4, 158.5)
  line L3 (4, 158.5) -> (4, 148.5)
  dimension "d953" = 4
  dimension "d954" = 148.5
  dimension "d955" = 10
  dimension "d956" = 10
  constraint horizontal L0
  constraint vertical L1
  constraint horizontal L2
  constraint vertical L3
  measures "d953" horizontal distance of origin L0.start
  measures "d954" vertical distance of origin L0.start
  measures "d955" horizontal distance of L0.start L0.end
  measures "d956" vertical distance of L0.end L1.end
extrude "AO2 connector and cable allowance" add sketch "AO2 connector and cable allowance sketch" along normal blind 6.5 separate body makes body 32 in component "17 Chamber sensor envelopes TBD"
ref_plane "WorkPlane4" through (0, 0, 16) normal (0, 0, 1) x (1, 0, 0) in component "17 Chamber sensor envelopes TBD"
sketch "ZE07-CO total envelope sketch" plane through (0, 0, 16) normal (0, 0, 1) x (1, 0, 0) in component "17 Chamber sensor envelopes TBD"
  line L0 (-32.4, 145) -> (-7, 145)
  line L1 (-7, 145) -> (-7, 167.4)
  line L2 (-7, 167.4) -> (-32.4, 167.4)
  line L3 (-32.4, 167.4) -> (-32.4, 145)
  dimension "d961" = 32.4
  dimension "d962" = 145
  dimension "d963" = 25.4
  dimension "d964" = 22.4
  constraint horizontal L0
  constraint vertical L1
  constraint horizontal L2
  constraint vertical L3
  measures "d961" horizontal distance of origin L0.start
  measures "d962" vertical distance of origin L0.start
  measures "d963" horizontal distance of L0.start L0.end
  measures "d964" vertical distance of L0.end L1.end
extrude "ZE07-CO total envelope" add sketch "ZE07-CO total envelope sketch" along normal blind 21.75 separate body makes body 33 in component "17 Chamber sensor envelopes TBD"
ref_plane "WorkPlane5" through (0, 0, 8) normal (0, 0, 1) x (1, 0, 0) in component "17 Chamber sensor envelopes TBD"
sketch "MD62 body envelope sketch" plane through (0, 0, 8) normal (0, 0, 1) x (1, 0, 0) in component "17 Chamber sensor envelopes TBD"
  line L0 (-26, 135) -> (-7, 135)
  line L1 (-7, 135) -> (-7, 144.5)
  line L2 (-7, 144.5) -> (-26, 144.5)
  line L3 (-26, 144.5) -> (-26, 135)
  dimension "d969" = 26
  dimension "d970" = 135
  dimension "d971" = 19
  dimension "d972" = 9.5
  constraint horizontal L0
  constraint vertical L1
  constraint horizontal L2
  constraint vertical L3
  measures "d969" horizontal distance of origin L0.start
  measures "d970" vertical distance of origin L0.start
  measures "d971" horizontal distance of L0.start L0.end
  measures "d972" vertical distance of L0.end L1.end
extrude "MD62 body envelope" add sketch "MD62 body envelope sketch" along normal blind 14 separate body makes body 34 in component "17 Chamber sensor envelopes TBD"
ref_plane "WorkPlane6" through (0, 0, 22) normal (0, 0, 1) x (1, 0, 0) in component "17 Chamber sensor envelopes TBD"
sketch "MD62 untrimmed lead allowance sketch" plane through (0, 0, 22) normal (0, 0, 1) x (1, 0, 0) in component "17 Chamber sensor envelopes TBD"
  line L0 (-26, 135) -> (-7, 135)
  line L1 (-7, 135) -> (-7, 144.5)
  line L2 (-7, 144.5) -> (-26, 144.5)
  line L3 (-26, 144.5) -> (-26, 135)
  dimension "d977" = 26
  dimension "d978" = 135
  dimension "d979" = 19
  dimension "d980" = 9.5
  constraint horizontal L0
  constraint vertical L1
  constraint horizontal L2
  constraint vertical L3
  measures "d977" horizontal distance of origin L0.start
  measures "d978" vertical distance of origin L0.start
  measures "d979" horizontal distance of L0.start L0.end
  measures "d980" vertical distance of L0.end L1.end
extrude "MD62 untrimmed lead allowance" add sketch "MD62 untrimmed lead allowance sketch" along normal blind 26 separate body makes body 35 in component "17 Chamber sensor envelopes TBD"
ref_plane "WorkPlane7" through (0, 0, 6.5) normal (0, 0, 1) x (1, 0, 0) in component "17 Chamber sensor envelopes TBD"
sketch "GYBMEP humidity module envelope TBD sketch" plane through (0, 0, 6.5) normal (0, 0, 1) x (1, 0, 0) in component "17 Chamber sensor envelopes TBD"
  line L0 (18, 145) -> (30, 145)
  line L1 (30, 145) -> (30, 162)
  line L2 (30, 162) -> (18, 162)
  line L3 (18, 162) -> (18, 145)
  dimension "d985" = 18
  dimension "d986" = 145
  dimension "d987" = 12
  dimension "d988" = 17
  constraint horizontal L0
  constraint vertical L1
  constraint horizontal L2
  constraint vertical L3
  measures "d985" horizontal distance of origin L0.start
  measures "d986" vertical distance of origin L0.start
  measures "d987" horizontal distance of L0.start L0.end
  measures "d988" vertical distance of L0.end L1.end
extrude "GYBMEP humidity module envelope TBD" add sketch "GYBMEP humidity module envelope TBD sketch" along normal blind 5 separate body makes body 36 in component "17 Chamber sensor envelopes TBD"
combine "Unite USB insert, backing flange and board supports" operation add target body 19 tool bodies 20 23 24 in component "14 Supported USB-C mounting insert TBD"
ref_plane "WorkPlane8" through (0, 0, 58.2) normal (0, 0, 1) x (1, 0, 0) in component "02 Single rear cover"
sketch "M3 head recess sketch" plane through (0, 0, 58.2) normal (0, 0, 1) x (1, 0, 0) in component "02 Single rear cover"
  circle A0 centre (-40, 8) radius 3
  dimension "d993" = 40
  dimension "d994" = 8
  dimension "d995" = 3
  measures "d993" horizontal distance of origin A0.centre
  measures "d994" vertical distance of origin A0.centre
  measures "d995" radius of A0
extrude "M3 head recess" cut sketch "M3 head recess sketch" along normal blind 1.9 bodies 2 in component "02 Single rear cover"
ref_plane "WorkPlane1" through (0, 0, 52) normal (0, 0, 1) x (1, 0, 0) in component "19 Rear M3 fastener envelopes TBD"
sketch "M3 heat-set insert envelope sketch" plane through (0, 0, 52) normal (0, 0, 1) x (1, 0, 0) in component "19 Rear M3 fastener envelopes TBD"
  circle A0 centre (-40, 8) radius 2.1
  dimension "d1000" = 40
  dimension "d1001" = 8
  dimension "d1002" = 2.1
  measures "d1000" horizontal distance of origin A0.centre
  measures "d1001" vertical distance of origin A0.centre
  measures "d1002" radius of A0
extrude "M3 heat-set insert envelope" add sketch "M3 heat-set insert envelope sketch" along normal blind 5 separate body makes body 37 in component "19 Rear M3 fastener envelopes TBD"
ref_plane "WorkPlane2" through (0, 0, 52) normal (0, 0, 1) x (1, 0, 0) in component "19 Rear M3 fastener envelopes TBD"
sketch "Insert thread clearance envelope sketch" plane through (0, 0, 52) normal (0, 0, 1) x (1, 0, 0) in component "19 Rear M3 fastener envelopes TBD"
  circle A0 centre (-40, 8) radius 1.55
  dimension "d1007" = 40
  dimension "d1008" = 8
  dimension "d1009" = 1.55
  measures "d1007" horizontal distance of origin A0.centre
  measures "d1008" vertical distance of origin A0.centre
  measures "d1009" radius of A0
extrude "Insert thread clearance envelope" cut sketch "Insert thread clearance envelope sketch" along normal blind 5 bodies 37 in component "19 Rear M3 fastener envelopes TBD"
ref_plane "WorkPlane3" through (0, 0, 54.2) normal (0, 0, 1) x (1, 0, 0) in component "19 Rear M3 fastener envelopes TBD"
sketch "M3 screw shaft envelope sketch" plane through (0, 0, 54.2) normal (0, 0, 1) x (1, 0, 0) in component "19 Rear M3 fastener envelopes TBD"
  circle A0 centre (-40, 8) radius 1.45
  dimension "d1014" = 40
  dimension "d1015" = 8
  dimension "d1016" = 1.45
  measures "d1014" horizontal distance of origin A0.centre
  measures "d1015" vertical distance of origin A0.centre
  measures "d1016" radius of A0
extrude "M3 screw shaft envelope" add sketch "M3 screw shaft envelope sketch" along normal blind 4 separate body makes body 38 in component "19 Rear M3 fastener envelopes TBD"
ref_plane "WorkPlane4" through (0, 0, 58.2) normal (0, 0, 1) x (1, 0, 0) in component "19 Rear M3 fastener envelopes TBD"
sketch "M3 low head envelope sketch" plane through (0, 0, 58.2) normal (0, 0, 1) x (1, 0, 0) in component "19 Rear M3 fastener envelopes TBD"
  circle A0 centre (-40, 8) radius 2.75
  dimension "d1021" = 40
  dimension "d1022" = 8
  dimension "d1023" = 2.75
  measures "d1021" horizontal distance of origin A0.centre
  measures "d1022" vertical distance of origin A0.centre
  measures "d1023" radius of A0
extrude "M3 low head envelope" add sketch "M3 low head envelope sketch" along normal blind 1.8 separate body makes body 39 in component "19 Rear M3 fastener envelopes TBD"
ref_plane "WorkPlane9" through (0, 0, 58.2) normal (0, 0, 1) x (1, 0, 0) in component "02 Single rear cover"
sketch "M3 head recess sketch (1)" plane through (0, 0, 58.2) normal (0, 0, 1) x (1, 0, 0) in component "02 Single rear cover"
  circle A0 centre (-40, 90) radius 3
  dimension "d1028" = 40
  dimension "d1029" = 90
  dimension "d1030" = 3
  measures "d1028" horizontal distance of origin A0.centre
  measures "d1029" vertical distance of origin A0.centre
  measures "d1030" radius of A0
extrude "M3 head recess (1)" cut sketch "M3 head recess sketch (1)" along normal blind 1.9 bodies 2 in component "02 Single rear cover"
ref_plane "WorkPlane5" through (0, 0, 52) normal (0, 0, 1) x (1, 0, 0) in component "19 Rear M3 fastener envelopes TBD"